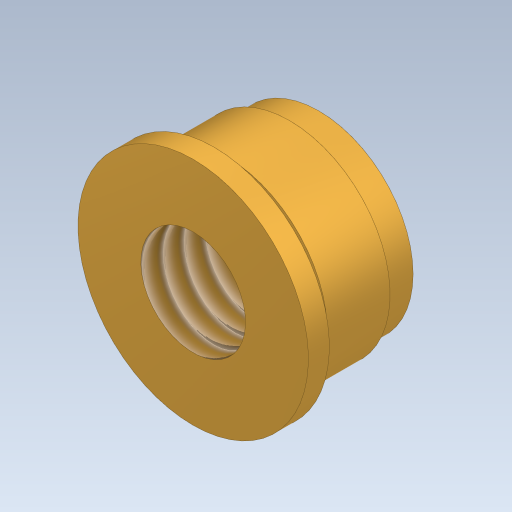
# Autodesk Inventor part: _FB-305530CD
Saved by Autodesk Inventor 2024 (Build 280153000, 153)
## iProperties
Created: 2023-10-01
Part Number: _FB-305530CD
Material: 真鍮、ソフト イエロー
Document SubType Name: Modeling
Designer: michi
Density: 8.47 g/cm^3
Appearance: 真鍮 - サテン
Author: michi
Autodesk Inventor part; units mm, degrees
ref_plane "YZ Plane" through (0, 0, 0) normal (1, 0, 0) x (0, 1, 0)
ref_plane "XZ Plane" through (0, 0, 0) normal (0, 1, 0) x (-1, 0, 0)
ref_plane "XY Plane" through (0, 0, 0) normal (0, 0, 1) x (1, 0, 0)
sketch "スケッチ1" plane through (0, 0, 0) normal (1, 0, 0) x (0, 1, 0)
  line L0 (2.75, 1.5) -> (1.25, 1.5)
  line L1 (1.25, 1.5) -> (1.25, 1)
  line L2 (1.25, 1) -> (2.75, 1)
  line L3 (2.75, 1) -> (2.75, 1.5)
  line L4 (2.25, 1) -> (1.25, 1)
  line L5 (1.25, 1) -> (1.25, -1.5)
  line L6 (1.25, -1.5) -> (2.25, -1.5)
  line L7 (2.25, -1.5) -> (2.25, 1)
  line L8 (0, 1.5) -> (0, -1.5) construction
  line L9 (2.25, 0.7) -> (2.4, 0.7)
  line L10 (2.4, 0.7) -> (2.4, -0.8)
  line L11 (2.4, -0.8) -> (2.25, -0.8)
  line L12 (2.25, -0.8) -> (2.25, 0.7)
  point P0 (0, 0)
  point P1 (0, 0)
  dimension "d0" = 3
  dimension "d1" = 5.5
  dimension "d2" = 4.5
  dimension "d3" = 0.5
  dimension "d4" = 2.5
  dimension "d8" = 4.8
  dimension "d9" = 0.3
  dimension "d10" = 1.5
  constraints: 26 end point, 6 parallel, 3 horizontal, 3 perpendicular, 3 point on line, 2 collinear, 1 coincident, 1 midpoint, 1 vertical
  measures "d0" distance between parallel lines of L6 L0
  measures "d1" diameter of L3 L8
  measures "d2" diameter of L7 L8
  measures "d3" distance of L2.end L0.start
  measures "d4" diameter of L5 L8
  measures "d8" diameter of L10 L8
  measures "d9" distance between parallel lines of L9 L4
  measures "d10" distance of L9.end L10.end
revolve "回転1" add sketch "スケッチ1" angle 360 about axis through (0, 0, 1.5) along (0, 0, -1)
thread "ねじ1" size "M3x0.5" class "6H" standard "ANSI Metric M Profile" length 30.3
